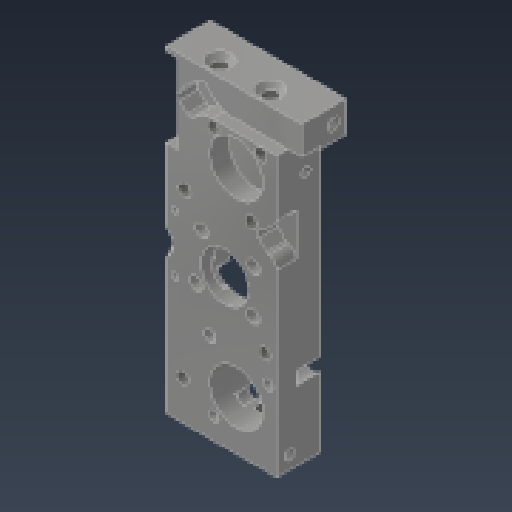
# Autodesk Inventor part: LeftGearbox
Saved by Autodesk Inventor 2027.1 (Build 311270010, 270A)
## iProperties
Created: 2026-04-13
Part Number: LeftGearbox
Material: Steel
Document SubType Name: Modeling
Designer: szymo
Density: 7.85 g/cm^3
Appearance: Nylon 6(1)
Mass: 68.9127 g
Surface Area: 68.8445 cm^2
Volume: 8.77869 cm^3
Author: szymo
Autodesk Inventor part; units mm, degrees
(part 1 of 2)
sketch "Sketch1" plane through (0, 0, 0) normal (0, 0, 1) x (1, 0, 0)
  circle A0 centre (14.75, -56.1789) radius 14.75 construction
  circle A1 centre (14.75, -56.1789) radius 14 construction
  circle A2 centre (14.75, -56.1789) radius 5.5
  circle A3 centre (14.7, -14.7) radius 5.5707
  circle A4 centre (14.7, -14.7) radius 14.7 construction
  circle A5 centre (12.35, -35.5681) radius 5
  circle A6 centre (9.3012, -47.7937) radius 8 construction
  circle A7 centre (9.3012, -47.7937) radius 4.2 construction
  circle A8 centre (12.35, -35.2722) radius 9.5572 construction
  line L0 (23.2, -66.4289) -> (0, -66.4289)
  line L1 (0, -66.4289) -> (0, 0)
  line L2 (0, 0) -> (23.2, 0)
  line L3 (23.2, 0) -> (23.2, -66.4289)
  circle A9 centre (12.35, -35.2722) radius 9.9572
  circle A10 centre (9.3012, -47.7937) radius 8.4
  line L4 (29.5, -56.1789) -> (23.2, -56.1789)
  line L5 (14.75, -56.1789) -> (23.2, -56.1789) construction
  line L6 (2.5, -8.5619) -> (2.3628, -10.4638) construction
  arc A11 (21.5927, -27.2496) -> (27.2496, -21.5927) centre (14.7, -14.7) ccw
  line L7 (27.2496, -21.5927) -> (24.0092, -18.3523)
  arc A12 (18.3523, -24.0092) -> (24.0092, -18.3523) centre (14.7, -14.7) ccw construction
  line L8 (18.3523, -24.0092) -> (21.5927, -27.2496)
  line L9 (18.3523, -24.0092) -> (24.0092, -18.3523)
  line L10 (23.2, -6.5) -> (28.4, -6.5)
  line L11 (28.4, -6.5) -> (28.4, 0)
  line L12 (28.4, 0) -> (23.2, 0)
  circle A13 centre (9.3012, -47.7937) radius 4.6
  circle A14 centre (14.75, -56.1789) radius 14.75 projected
  circle A15 centre (14.75, -56.1789) radius 14.25 projected
  circle A16 centre (9.0931, -61.8357) radius 1.0564 projected
  circle A17 centre (20.4069, -50.522) radius 1.0564 projected
  circle A18 centre (14.75, -56.1789) radius 5.5 projected
  circle A19 centre (14.75, -56.1789) radius 14.25 projected
  circle A20 centre (14.75, -14.75) radius 14.75 projected
  circle A21 centre (14.75, -14.75) radius 14.25 projected
  circle A22 centre (14.75, -14.75) radius 5.5 projected
  arc A23 (9.8338, -26.3037) -> (9.7739, -27.7306) centre (15.759, -27.2671) ccw projected
  arc A24 (10.3221, -26.1847) -> (9.8338, -26.3037) centre (12.35, -35.5681) ccw projected
  arc A25 (11.0317, -27.4241) -> (10.3221, -26.1847) centre (5.5043, -29.766) ccw projected
  arc A26 (11.4597, -27.3663) -> (11.0317, -27.4241) centre (12.35, -35.5681) ccw projected
  arc A27 (11.815, -25.983) -> (11.4597, -27.3663) centre (17.4104, -28.1572) ccw projected
  arc A28 (12.3173, -25.9682) -> (11.815, -25.983) centre (12.35, -35.5681) ccw projected
  arc A29 (12.7537, -27.328) -> (12.3173, -25.9682) centre (6.8602, -28.4694) ccw projected
  arc A30 (13.1844, -27.3604) -> (12.7537, -27.328) centre (12.35, -35.5681) ccw projected
  arc A31 (13.8195, -26.0813) -> (13.1844, -27.3604) centre (18.8407, -29.3713) ccw projected
  arc A32 (14.314, -26.1712) -> (13.8195, -26.0813) centre (12.35, -35.5681) ccw projected
  arc A33 (14.4581, -27.592) -> (14.314, -26.1712) centre (8.4561, -27.4832) ccw projected
  arc A34 (14.8727, -27.7133) -> (14.4581, -27.592) centre (12.35, -35.5681) ccw projected
  arc A35 (15.7598, -26.5941) -> (14.8727, -27.7133) centre (19.9872, -30.8562) ccw projected
  arc A36 (16.2248, -26.7848) -> (15.7598, -26.5941) centre (12.35, -35.5681) ccw projected
  arc A37 (16.0704, -28.2046) -> (16.2248, -26.7848) centre (10.2221, -26.8502) ccw projected
  arc A38 (16.4507, -28.4094) -> (16.0704, -28.2046) centre (12.35, -35.5681) ccw projected
  arc A39 (17.5511, -27.4991) -> (16.4507, -28.4094) centre (20.8, -32.547) ccw projected
  arc A40 (17.9663, -27.7824) -> (17.5511, -27.4991) centre (12.35, -35.5681) ccw projected
  arc A41 (17.52, -29.139) -> (17.9663, -27.7824) centre (12.0812, -26.5983) ccw projected
  arc A42 (17.8494, -29.4184) -> (17.52, -29.139) centre (12.35, -35.5681) ccw projected
  arc A43 (19.1151, -28.7568) -> (17.8494, -29.4184) centre (21.2434, -34.3699) ccw projected
  arc A44 (19.4623, -29.1202) -> (19.1151, -28.7568) centre (12.35, -35.5681) ccw projected
  arc A45 (18.7437, -30.3544) -> (19.4623, -29.1202) centre (13.952, -26.7385) ccw projected
  arc A46 (19.0078, -30.6962) -> (18.7437, -30.3544) centre (12.35, -35.5681) ccw projected
  arc A47 (20.3834, -30.3122) -> (19.0078, -30.6962) centre (21.2982, -36.2451) ccw projected
  arc A48 (20.6475, -30.7399) -> (20.3834, -30.3122) centre (12.35, -35.5681) ccw projected
  arc A49 (19.688, -31.7977) -> (20.6475, -30.7399) centre (15.7527, -27.2645) ccw projected
  arc A50 (19.8753, -32.1869) -> (19.688, -31.7977) centre (12.35, -35.5681) ccw projected
  arc A51 (21.3006, -32.0973) -> (19.8753, -32.1869) centre (20.9619, -38.0908) ccw projected
  arc A52 (21.47, -32.5705) -> (21.3006, -32.0973) centre (12.35, -35.5681) ccw projected
  arc A53 (20.3116, -33.4058) -> (21.47, -32.5705) centre (17.4048, -28.1534) ccw projected
  arc A54 (20.4138, -33.8254) -> (20.3116, -33.4058) centre (12.35, -35.5681) ccw projected
  arc A55 (21.8266, -34.0341) -> (20.4138, -33.8254) centre (20.2492, -39.8262) ccw projected
  arc A56 (21.8939, -34.5322) -> (21.8266, -34.0341) centre (12.35, -35.5681) ccw projected
  arc A57 (20.5872, -35.1083) -> (21.8939, -34.5322) centre (18.836, -29.3664) ccw projected
  arc A58 (20.6, -35.54) -> (20.5872, -35.1083) centre (12.35, -35.5681) ccw projected
  arc A59 (21.9385, -36.0379) -> (20.6, -35.54) centre (19.1913, -41.3755) ccw projected
  arc A60 (21.9008, -36.5391) -> (21.9385, -36.0379) centre (12.35, -35.5681) ccw projected
  arc A61 (20.5028, -36.831) -> (21.9008, -36.5391) centre (19.9836, -30.8504) ccw projected
  arc A62 (20.4255, -37.2559) -> (20.5028, -36.831) centre (12.35, -35.5681) ccw projected
  arc A63 (21.6313, -38.0212) -> (20.4255, -37.2559) centre (17.8344, -42.671) ccw projected
  arc A64 (21.4902, -38.5036) -> (21.6313, -38.0212) centre (12.35, -35.5681) ccw projected
  arc A65 (20.0621, -38.4984) -> (21.4902, -38.5036) centre (20.7977, -32.5406) ccw projected
  arc A66 (19.8981, -38.898) -> (20.0621, -38.4984) centre (12.35, -35.5681) ccw projected
  arc A67 (20.9184, -39.8973) -> (19.8981, -38.898) centre (16.2378, -43.656) ccw projected
  arc A68 (20.6801, -40.3398) -> (20.9184, -39.8973) centre (12.35, -35.5681) ccw projected
  arc A69 (19.2843, -40.0378) -> (20.6801, -40.3398) centre (21.2425, -34.3632) ccw projected
  arc A70 (19.0409, -40.3946) -> (19.2843, -40.0378) centre (12.35, -35.5681) ccw projected
  arc A71 (19.8311, -41.5842) -> (19.0409, -40.3946) centre (14.4713, -44.2876) ccw projected
  arc A72 (19.506, -41.9675) -> (19.8311, -41.5842) centre (12.35, -35.5681) ccw projected
  arc A73 (18.2034, -41.3819) -> (19.506, -41.9675) centre (21.2987, -36.2383) ccw projected
  arc A74 (17.8912, -41.6802) -> (18.2034, -41.3819) centre (12.35, -35.5681) ccw projected
  arc A75 (18.4168, -43.0081) -> (17.8912, -41.6802) centre (12.612, -44.5381) ccw projected
  arc A76 (18.0191, -43.3154) -> (18.4168, -43.0081) centre (12.35, -35.5681) ccw projected
  arc A77 (16.8668, -42.4718) -> (18.0191, -43.3154) centre (20.9638, -38.0842) ccw projected
  arc A78 (16.4993, -42.6987) -> (16.8668, -42.4718) centre (12.35, -35.5681) ccw projected
  arc A79 (16.7374, -44.1069) -> (16.4993, -42.6987) centre (10.7413, -44.3966) ccw projected
  arc A80 (16.2845, -44.3248) -> (16.7374, -44.1069) centre (12.35, -35.5681) ccw projected
  arc A81 (15.3327, -43.26) -> (16.2845, -44.3248) centre (20.2525, -39.8202) ccw projected
  arc A82 (14.9261, -43.4056) -> (15.3327, -43.26) centre (12.35, -35.5681) ccw projected
  arc A83 (14.8662, -44.8325) -> (14.9261, -43.4056) centre (8.941, -43.8692) ccw projected
  arc A84 (14.3779, -44.9515) -> (14.8662, -44.8325) centre (12.35, -35.5681) ccw projected
  arc A85 (13.6683, -43.7121) -> (14.3779, -44.9515) centre (19.1957, -41.3703) ccw projected
  arc A86 (13.2403, -43.7699) -> (13.6683, -43.7121) centre (12.35, -35.5681) ccw projected
  arc A87 (12.885, -45.1532) -> (13.2403, -43.7699) centre (7.2896, -42.979) ccw projected
  arc A88 (12.3827, -45.1681) -> (12.885, -45.1532) centre (12.35, -35.5681) ccw projected
  arc A89 (11.9463, -43.8082) -> (12.3827, -45.1681) centre (17.8398, -42.6668) ccw projected
  arc A90 (11.5156, -43.7758) -> (11.9463, -43.8082) centre (12.35, -35.5681) ccw projected
  arc A91 (10.8805, -45.055) -> (11.5156, -43.7758) centre (5.8593, -41.7649) ccw projected
  arc A92 (10.386, -44.9651) -> (10.8805, -45.055) centre (12.35, -35.5681) ccw projected
  arc A93 (10.2419, -43.5442) -> (10.386, -44.9651) centre (16.2439, -43.6531) ccw projected
  arc A94 (9.8273, -43.423) -> (10.2419, -43.5442) centre (12.35, -35.5681) ccw projected
  arc A95 (8.9402, -44.5421) -> (9.8273, -43.423) centre (4.7128, -40.28) ccw projected
  arc A96 (8.4752, -44.3514) -> (8.9402, -44.5421) centre (12.35, -35.5681) ccw projected
  arc A97 (8.6296, -42.9316) -> (8.4752, -44.3514) centre (14.4779, -44.286) ccw projected
  arc A98 (8.2493, -42.7268) -> (8.6296, -42.9316) centre (12.35, -35.5681) ccw projected
  arc A99 (7.1489, -43.6371) -> (8.2493, -42.7268) centre (3.9, -38.5892) ccw projected
  arc A100 (6.7337, -43.3538) -> (7.1489, -43.6371) centre (12.35, -35.5681) ccw projected
  arc A101 (7.18, -41.9972) -> (6.7337, -43.3538) centre (12.6188, -44.5379) ccw projected
  arc A102 (6.8506, -41.7178) -> (7.18, -41.9972) centre (12.35, -35.5681) ccw projected
  arc A103 (5.5849, -42.3794) -> (6.8506, -41.7178) centre (3.4566, -36.7663) ccw projected
  arc A104 (5.2377, -42.016) -> (5.5849, -42.3794) centre (12.35, -35.5681) ccw projected
  arc A105 (5.9563, -40.7818) -> (5.2377, -42.016) centre (10.748, -44.3978) ccw projected
  arc A106 (5.6922, -40.44) -> (5.9563, -40.7818) centre (12.35, -35.5681) ccw projected
  arc A107 (4.3166, -40.824) -> (5.6922, -40.44) centre (3.4018, -34.8911) ccw projected
  arc A108 (4.0525, -40.3964) -> (4.3166, -40.824) centre (12.35, -35.5681) ccw projected
  arc A109 (5.012, -39.3385) -> (4.0525, -40.3964) centre (8.9473, -43.8718) ccw projected
  arc A110 (4.8247, -38.9493) -> (5.012, -39.3385) centre (12.35, -35.5681) ccw projected
  arc A111 (3.3994, -39.0389) -> (4.8247, -38.9493) centre (3.7381, -33.0454) ccw projected
  arc A112 (3.23, -38.5657) -> (3.3994, -39.0389) centre (12.35, -35.5681) ccw projected
  arc A113 (4.3884, -37.7305) -> (3.23, -38.5657) centre (7.2952, -42.9828) ccw projected
  arc A114 (4.2862, -37.3108) -> (4.3884, -37.7305) centre (12.35, -35.5681) ccw projected
  arc A115 (2.8734, -37.1021) -> (4.2862, -37.3108) centre (4.4508, -31.31) ccw projected
  arc A116 (2.8061, -36.6041) -> (2.8734, -37.1021) centre (12.35, -35.5681) ccw projected
  arc A117 (4.1128, -36.0279) -> (2.8061, -36.6041) centre (5.864, -41.7699) ccw projected
  arc A118 (4.1, -35.5962) -> (4.1128, -36.0279) centre (12.35, -35.5681) ccw projected
  arc A119 (2.7615, -35.0983) -> (4.1, -35.5962) centre (5.5087, -29.7608) ccw projected
  arc A120 (2.7992, -34.5971) -> (2.7615, -35.0983) centre (12.35, -35.5681) ccw projected
  arc A121 (4.1972, -34.3053) -> (2.7992, -34.5971) centre (4.7164, -40.2858) ccw projected
  arc A122 (4.2745, -33.8803) -> (4.1972, -34.3053) centre (12.35, -35.5681) ccw projected
  arc A123 (3.0687, -33.115) -> (4.2745, -33.8803) centre (6.8656, -28.4653) ccw projected
  arc A124 (3.2098, -32.6326) -> (3.0687, -33.115) centre (12.35, -35.5681) ccw projected
  arc A125 (4.6379, -32.6378) -> (3.2098, -32.6326) centre (3.9023, -38.5956) ccw projected
  arc A126 (4.8019, -32.2382) -> (4.6379, -32.6378) centre (12.35, -35.5681) ccw projected
  arc A127 (3.7816, -31.2389) -> (4.8019, -32.2382) centre (8.4622, -27.4802) ccw projected
  arc A128 (4.0199, -30.7964) -> (3.7816, -31.2389) centre (12.35, -35.5681) ccw projected
  arc A129 (5.4157, -31.0984) -> (4.0199, -30.7964) centre (3.4575, -36.7731) ccw projected
  arc A130 (5.6591, -30.7416) -> (5.4157, -31.0984) centre (12.35, -35.5681) ccw projected
  arc A131 (4.8689, -29.5521) -> (5.6591, -30.7416) centre (10.2287, -26.8486) ccw projected
  arc A132 (5.194, -29.1688) -> (4.8689, -29.5521) centre (12.35, -35.5681) ccw projected
  arc A133 (6.4966, -29.7544) -> (5.194, -29.1688) centre (3.4013, -34.8979) ccw projected
  arc A134 (6.8088, -29.456) -> (6.4966, -29.7544) centre (12.35, -35.5681) ccw projected
  arc A135 (6.2832, -28.1281) -> (6.8088, -29.456) centre (12.088, -26.5981) ccw projected
  arc A136 (6.6809, -27.8208) -> (6.2832, -28.1281) centre (12.35, -35.5681) ccw projected
  arc A137 (7.8332, -28.6644) -> (6.6809, -27.8208) centre (3.7362, -33.052) ccw projected
  arc A138 (8.2007, -28.4375) -> (7.8332, -28.6644) centre (12.35, -35.5681) ccw projected
  arc A139 (7.9626, -27.0293) -> (8.2007, -28.4375) centre (13.9587, -26.7397) ccw projected
  arc A140 (8.4155, -26.8114) -> (7.9626, -27.0293) centre (12.35, -35.5681) ccw projected
  arc A141 (9.3673, -27.8762) -> (8.4155, -26.8114) centre (4.4475, -31.316) ccw projected
  arc A142 (9.7739, -27.7306) -> (9.3673, -27.8762) centre (12.35, -35.5681) ccw projected
  circle A143 centre (9.3012, -47.7937) radius 1.25 projected
  arc A144 (9.6251, -54.6611) -> (10.0958, -55.7541) centre (14.4225, -53.2431) ccw projected
  arc A145 (9.2653, -54.6686) -> (9.6251, -54.6611) centre (9.3012, -47.7937) ccw projected
  arc A146 (8.8408, -55.7804) -> (9.2653, -54.6686) centre (4.4127, -53.4528) ccw projected
  arc A147 (8.4234, -55.7454) -> (8.8408, -55.7804) centre (9.3012, -47.7937) ccw projected
  arc A148 (8.1902, -54.5783) -> (8.4234, -55.7454) centre (13.1776, -54.1888) ccw projected
  arc A149 (7.8367, -54.5109) -> (8.1902, -54.5783) centre (9.3012, -47.7937) ccw projected
  arc A150 (7.1903, -55.5102) -> (7.8367, -54.5109) centre (3.3429, -52.3128) ccw projected
  arc A151 (6.7893, -55.3891) -> (7.1903, -55.5102) centre (9.3012, -47.7937) ccw projected
  arc A152 (6.8039, -54.1991) -> (6.7893, -55.3891) centre (11.7633, -54.855) ccw projected
  arc A153 (6.4721, -54.0596) -> (6.8039, -54.1991) centre (9.3012, -47.7937) ccw projected
  arc A154 (5.6321, -54.9027) -> (6.4721, -54.0596) centre (2.5336, -50.9752) ccw projected
  arc A155 (5.265, -54.7009) -> (5.6321, -54.9027) centre (9.3012, -47.7937) ccw projected
  arc A156 (5.5267, -53.5399) -> (5.265, -54.7009) centre (10.2414, -55.2125) ccw projected
  arc A157 (5.2312, -53.3345) -> (5.5267, -53.5399) centre (9.3012, -47.7937) ccw projected
  arc A158 (4.2342, -53.9845) -> (5.2312, -53.3345) centre (2.02, -49.4986) ccw projected
  arc A159 (3.9172, -53.7108) -> (4.2342, -53.9845) centre (9.3012, -47.7937) ccw projected
  arc A160 (4.4145, -52.6296) -> (3.9172, -53.7108) centre (8.6783, -55.2459) ccw projected
  arc A161 (4.1681, -52.3672) -> (4.4145, -52.6296) centre (9.3012, -47.7937) ccw projected
  arc A162 (3.0578, -52.7957) -> (4.1681, -52.3672) centre (1.8246, -47.9475) ccw projected
  arc A163 (2.8046, -52.4621) -> (3.0578, -52.7957) centre (9.3012, -47.7937) ccw projected
  arc A164 (3.5159, -51.5079) -> (2.8046, -52.4621) centre (7.1426, -54.9535) ccw projected
  arc A165 (3.3294, -51.2) -> (3.5159, -51.5079) centre (9.3012, -47.7937) ccw projected
  arc A166 (2.1543, -51.3883) -> (3.3294, -51.2) centre (1.956, -46.3897) ccw projected
  arc A167 (1.9759, -51.0093) -> (2.1543, -51.3883) centre (9.3012, -47.7937) ccw projected
  arc A168 (2.8701, -50.2239) -> (1.9759, -51.0093) centre (5.7011, -54.3483) ccw projected
  arc A169 (2.7517, -49.884) -> (2.8701, -50.2239) centre (9.3012, -47.7937) ccw projected
  arc A170 (1.5631, -49.8238) -> (2.7517, -49.884) centre (2.4085, -44.8932) ccw projected
  arc A171 (1.4674, -49.4161) -> (1.5631, -49.8238) centre (9.3012, -47.7937) ccw projected
  arc A172 (2.5053, -48.8337) -> (1.4674, -49.4161) centre (4.417, -53.4565) ccw projected
  arc A173 (2.4602, -48.4766) -> (2.5053, -48.8337) centre (9.3012, -47.7937) ccw projected
  arc A174 (1.3101, -48.1706) -> (2.4602, -48.4766) centre (3.1621, -43.5235) ccw projected
  arc A175 (1.3013, -47.7519) -> (1.3101, -48.1706) centre (9.3012, -47.7937) ccw projected
  arc A176 (2.4376, -47.398) -> (1.3013, -47.7519) centre (3.3464, -52.3173) ccw projected
  arc A177 (2.4677, -47.0393) -> (2.4376, -47.398) centre (9.3012, -47.7937) ccw projected
  arc A178 (1.4064, -46.5009) -> (2.4677, -47.0393) centre (4.1841, -42.3404) ccw projected
  arc A179 (1.4848, -46.0895) -> (1.4064, -46.5009) centre (9.3012, -47.7937) ccw projected
  arc A180 (2.6699, -45.9796) -> (1.4848, -46.0895) centre (2.536, -50.9804) ccw projected
  arc A181 (2.7739, -45.635) -> (2.6699, -45.9796) centre (9.3012, -47.7937) ccw projected
  arc A182 (1.8477, -44.8877) -> (2.7739, -45.635) centre (5.4297, -41.3957) ccw projected
  arc A183 (2.01, -44.5016) -> (1.8477, -44.8877) centre (9.3012, -47.7937) ccw projected
  arc A184 (3.192, -44.6405) -> (2.01, -44.5016) centre (2.0213, -49.5042) ccw projected
  arc A185 (3.3653, -44.3251) -> (3.192, -44.6405) centre (9.3012, -47.7937) ccw projected
  arc A186 (2.6147, -43.4016) -> (3.3653, -44.3251) centre (6.8445, -40.7306) ccw projected
  arc A187 (2.8538, -43.0576) -> (2.6147, -43.4016) centre (9.3012, -47.7937) ccw projected
  arc A188 (3.981, -43.4392) -> (2.8538, -43.0576) centre (1.8248, -47.9532) ccw projected
  arc A189 (4.2162, -43.1668) -> (3.981, -43.4392) centre (9.3012, -47.7937) ccw projected
  arc A190 (3.674, -42.1073) -> (4.2162, -43.1668) centre (8.3667, -40.3741) ccw projected
  arc A191 (3.9793, -41.8206) -> (3.674, -42.1073) centre (9.3012, -47.7937) ccw projected
  arc A192 (5.0026, -42.4283) -> (3.9793, -41.8206) centre (1.955, -46.3953) ccw projected
  arc A193 (5.2893, -42.2107) -> (5.0026, -42.4283) centre (9.3012, -47.7937) ccw projected
  arc A194 (4.9792, -41.0616) -> (5.2893, -42.2107) centre (9.9298, -40.342) ccw projected
  arc A195 (5.3375, -40.8447) -> (4.9792, -41.0616) centre (9.3012, -47.7937) ccw projected
  arc A196 (6.2121, -41.6518) -> (5.3375, -40.8447) centre (2.4062, -44.8985) ccw projected
  arc A197 (6.5378, -41.4985) -> (6.2121, -41.6518) centre (9.3012, -47.7937) ccw projected
  arc A198 (6.4734, -40.3102) -> (6.5378, -41.4985) centre (11.4653, -40.6355) ccw projected
  arc A199 (6.8689, -40.1724) -> (6.4734, -40.3102) centre (9.3012, -47.7937) ccw projected
  arc A200 (7.5566, -41.1437) -> (6.8689, -40.1724) centre (3.1589, -43.5282) ccw projected
  arc A201 (7.907, -41.0616) -> (7.5566, -41.1437) centre (9.3012, -47.7937) ccw projected
  arc A202 (8.0911, -39.8858) -> (7.907, -41.0616) centre (12.9063, -41.2419) ccw projected
  arc A203 (8.5066, -39.8333) -> (8.0911, -39.8858) centre (9.3012, -47.7937) ccw projected
  arc A204 (8.9773, -40.9263) -> (8.5066, -39.8333) centre (4.18, -42.3443) ccw projected
  arc A205 (9.3372, -40.9188) -> (8.9773, -40.9263) centre (9.3012, -47.7937) ccw projected
  arc A206 (9.7617, -39.807) -> (9.3372, -40.9188) centre (14.1897, -42.1346) ccw projected
  arc A207 (10.179, -39.842) -> (9.7617, -39.807) centre (9.3012, -47.7937) ccw projected
  arc A208 (10.4122, -41.0091) -> (10.179, -39.842) centre (5.4249, -41.3986) ccw projected
  arc A209 (10.7658, -41.0765) -> (10.4122, -41.0091) centre (9.3012, -47.7937) ccw projected
  arc A210 (11.4121, -40.0772) -> (10.7658, -41.0765) centre (15.2595, -43.2746) ccw projected
  arc A211 (11.8131, -40.1983) -> (11.4121, -40.0772) centre (9.3012, -47.7937) ccw projected
  arc A212 (11.7985, -41.3883) -> (11.8131, -40.1983) centre (6.8392, -40.7324) ccw projected
  arc A213 (12.1303, -41.5278) -> (11.7985, -41.3883) centre (9.3012, -47.7937) ccw projected
  arc A214 (12.9704, -40.6847) -> (12.1303, -41.5278) centre (16.0689, -44.6122) ccw projected
  arc A215 (13.3374, -40.8865) -> (12.9704, -40.6847) centre (9.3012, -47.7937) ccw projected
  arc A216 (13.0757, -42.0475) -> (13.3374, -40.8865) centre (8.3611, -40.3749) ccw projected
  arc A217 (13.3713, -42.2529) -> (13.0757, -42.0475) centre (9.3012, -47.7937) ccw projected
  arc A218 (14.3682, -41.6029) -> (13.3713, -42.2529) centre (16.5824, -46.0888) ccw projected
  arc A219 (14.6853, -41.8766) -> (14.3682, -41.6029) centre (9.3012, -47.7937) ccw projected
  arc A220 (14.1879, -42.9578) -> (14.6853, -41.8766) centre (9.9241, -40.3415) ccw projected
  arc A221 (14.4343, -43.2202) -> (14.1879, -42.9578) centre (9.3012, -47.7937) ccw projected
  arc A222 (15.5446, -42.7917) -> (14.4343, -43.2202) centre (16.7778, -47.6399) ccw projected
  arc A223 (15.7979, -43.1253) -> (15.5446, -42.7917) centre (9.3012, -47.7937) ccw projected
  arc A224 (15.0866, -44.0795) -> (15.7979, -43.1253) centre (11.4599, -40.6339) ccw projected
  arc A225 (15.273, -44.3874) -> (15.0866, -44.0795) centre (9.3012, -47.7937) ccw projected
  arc A226 (16.4482, -44.1991) -> (15.273, -44.3874) centre (16.6464, -49.1977) ccw projected
  arc A227 (16.6265, -44.5781) -> (16.4482, -44.1991) centre (9.3012, -47.7937) ccw projected
  arc A228 (15.7324, -45.3635) -> (16.6265, -44.5781) centre (12.9013, -41.2391) ccw projected
  arc A229 (15.8508, -45.7034) -> (15.7324, -45.3635) centre (9.3012, -47.7937) ccw projected
  arc A230 (17.0393, -45.7636) -> (15.8508, -45.7034) centre (16.194, -50.6942) ccw projected
  arc A231 (17.135, -46.1713) -> (17.0393, -45.7636) centre (9.3012, -47.7937) ccw projected
  arc A232 (16.0971, -46.7537) -> (17.135, -46.1713) centre (14.1854, -42.1309) ccw projected
  arc A233 (16.1422, -47.1108) -> (16.0971, -46.7537) centre (9.3012, -47.7937) ccw projected
  arc A234 (17.2923, -47.4168) -> (16.1422, -47.1108) centre (15.4403, -52.0639) ccw projected
  arc A235 (17.3011, -47.8355) -> (17.2923, -47.4168) centre (9.3012, -47.7937) ccw projected
  arc A236 (16.1648, -48.1894) -> (17.3011, -47.8355) centre (15.2561, -43.2701) ccw projected
  arc A237 (16.1347, -48.5481) -> (16.1648, -48.1894) centre (9.3012, -47.7937) ccw projected
  arc A238 (17.1961, -49.0865) -> (16.1347, -48.5481) centre (14.4183, -53.247) ccw projected
  arc A239 (17.1176, -49.4979) -> (17.1961, -49.0865) centre (9.3012, -47.7937) ccw projected
  arc A240 (15.9326, -49.6078) -> (17.1176, -49.4979) centre (16.0664, -44.607) ccw projected
  arc A241 (15.8285, -49.9524) -> (15.9326, -49.6078) centre (9.3012, -47.7937) ccw projected
  arc A242 (16.7548, -50.6997) -> (15.8285, -49.9524) centre (13.1727, -54.1917) ccw projected
  arc A243 (16.5925, -51.0858) -> (16.7548, -50.6997) centre (9.3012, -47.7937) ccw projected
  arc A244 (15.4105, -50.9469) -> (16.5925, -51.0858) centre (16.5811, -46.0832) ccw projected
  arc A245 (15.2371, -51.2623) -> (15.4105, -50.9469) centre (9.3012, -47.7937) ccw projected
  arc A246 (15.9877, -52.1858) -> (15.2371, -51.2623) centre (11.7579, -54.8568) ccw projected
  arc A247 (15.7487, -52.5298) -> (15.9877, -52.1858) centre (9.3012, -47.7937) ccw projected
  arc A248 (14.6214, -52.1482) -> (15.7487, -52.5298) centre (16.7777, -47.6342) ccw projected
  arc A249 (14.3862, -52.4206) -> (14.6214, -52.1482) centre (9.3012, -47.7937) ccw projected
  arc A250 (14.9284, -53.4801) -> (14.3862, -52.4206) centre (10.2357, -55.2133) ccw projected
  arc A251 (14.6231, -53.7668) -> (14.9284, -53.4801) centre (9.3012, -47.7937) ccw projected
  arc A252 (13.5998, -53.1591) -> (14.6231, -53.7668) centre (16.6475, -49.1921) ccw projected
  arc A253 (13.3131, -53.3767) -> (13.5998, -53.1591) centre (9.3012, -47.7937) ccw projected
  arc A254 (13.6232, -54.5258) -> (13.3131, -53.3767) centre (8.6727, -55.2454) ccw projected
  arc A255 (13.2649, -54.7427) -> (13.6232, -54.5258) centre (9.3012, -47.7937) ccw projected
  arc A256 (12.3903, -53.9356) -> (13.2649, -54.7427) centre (16.1962, -50.6889) ccw projected
  arc A257 (12.0647, -54.0889) -> (12.3903, -53.9356) centre (9.3012, -47.7937) ccw projected
  arc A258 (12.1291, -55.2772) -> (12.0647, -54.0889) centre (7.1371, -54.9519) ccw projected
  arc A259 (11.7335, -55.415) -> (12.1291, -55.2772) centre (9.3012, -47.7937) ccw projected
  arc A260 (11.0459, -54.4437) -> (11.7335, -55.415) centre (15.4436, -52.0592) ccw projected
  arc A261 (10.6954, -54.5258) -> (11.0459, -54.4437) centre (9.3012, -47.7937) ccw projected
  arc A262 (10.5114, -55.7016) -> (10.6954, -54.5258) centre (5.6961, -54.3455) ccw projected
  arc A263 (10.0958, -55.7541) -> (10.5114, -55.7016) centre (9.3012, -47.7937) ccw projected
  circle A264 centre (9.3012, -47.7937) radius 1.25 projected
  arc A265 (10.3711, -45.1522) -> (10.3563, -43.7284) centre (6.7284, -44.4781) ccw projected
  arc A266 (10.7068, -45.3144) -> (10.3711, -45.1522) centre (9.3012, -47.7937) ccw projected
  arc A267 (11.8317, -44.4416) -> (10.7068, -45.3144) centre (13.4977, -47.7504) ccw projected
  arc A268 (12.2476, -44.8006) -> (11.8317, -44.4416) centre (9.3012, -47.7937) ccw projected
  arc A269 (11.5486, -46.041) -> (12.2476, -44.8006) centre (8.7309, -43.6359) ccw projected
  arc A270 (11.7581, -46.3493) -> (11.5486, -46.041) centre (9.3012, -47.7937) ccw projected
  arc A271 (13.1688, -46.156) -> (11.7581, -46.3493) centre (12.9572, -49.8545) ccw projected
  arc A272 (13.3494, -46.6748) -> (13.1688, -46.156) centre (9.3012, -47.7937) ccw projected
  arc A273 (12.1238, -47.3995) -> (13.3494, -46.6748) centre (10.8863, -43.9078) ccw projected
  arc A274 (12.1511, -47.7713) -> (12.1238, -47.3995) centre (9.3012, -47.7937) ccw projected
  arc A275 (13.4695, -48.3092) -> (12.1511, -47.7713) centre (11.437, -51.4064) ccw projected
  arc A276 (13.3665, -48.8488) -> (13.4695, -48.3092) centre (9.3012, -47.7937) ccw projected
  arc A277 (11.9428, -48.8636) -> (13.3665, -48.8488) centre (12.6169, -45.2209) ccw projected
  arc A278 (11.7805, -49.1993) -> (11.9428, -48.8636) centre (9.3012, -47.7937) ccw projected
  arc A279 (12.6533, -50.3242) -> (11.7805, -49.1993) centre (9.3445, -51.9902) ccw projected
  arc A280 (12.2943, -50.7401) -> (12.6533, -50.3242) centre (9.3012, -47.7937) ccw projected
  arc A281 (11.0539, -50.041) -> (12.2943, -50.7401) centre (13.459, -47.2234) ccw projected
  arc A282 (10.7456, -50.2506) -> (11.0539, -50.041) centre (9.3012, -47.7937) ccw projected
  arc A283 (10.9389, -51.6612) -> (10.7456, -50.2506) centre (7.2404, -51.4496) ccw projected
  arc A284 (10.4201, -51.8419) -> (10.9389, -51.6612) centre (9.3012, -47.7937) ccw projected
  arc A285 (9.6954, -50.6163) -> (10.4201, -51.8419) centre (13.1871, -49.3787) ccw projected
  arc A286 (9.3236, -50.6436) -> (9.6954, -50.6163) centre (9.3012, -47.7937) ccw projected
  arc A287 (8.7858, -51.9619) -> (9.3236, -50.6436) centre (5.6886, -49.9294) ccw projected
  arc A288 (8.2461, -51.859) -> (8.7858, -51.9619) centre (9.3012, -47.7937) ccw projected
  arc A289 (8.2313, -50.4352) -> (8.2461, -51.859) centre (11.874, -51.1093) ccw projected
  arc A290 (7.8957, -50.273) -> (8.2313, -50.4352) centre (9.3012, -47.7937) ccw projected
  arc A291 (6.7707, -51.1458) -> (7.8957, -50.273) centre (5.1047, -47.837) ccw projected
  arc A292 (6.3548, -50.7868) -> (6.7707, -51.1458) centre (9.3012, -47.7937) ccw projected
  arc A293 (7.0539, -49.5464) -> (6.3548, -50.7868) centre (9.8715, -51.9515) ccw projected
  arc A294 (6.8443, -49.2381) -> (7.0539, -49.5464) centre (9.3012, -47.7937) ccw projected
  arc A295 (5.4337, -49.4314) -> (6.8443, -49.2381) centre (5.6453, -45.7329) ccw projected
  arc A296 (5.253, -48.9126) -> (5.4337, -49.4314) centre (9.3012, -47.7937) ccw projected
  arc A297 (6.4786, -48.1879) -> (5.253, -48.9126) centre (7.7162, -51.6796) ccw projected
  arc A298 (6.4513, -47.8161) -> (6.4786, -48.1879) centre (9.3012, -47.7937) ccw projected
  arc A299 (5.133, -47.2782) -> (6.4513, -47.8161) centre (7.1655, -44.181) ccw projected
  arc A300 (5.2359, -46.7386) -> (5.133, -47.2782) centre (9.3012, -47.7937) ccw projected
  arc A301 (6.6597, -46.7238) -> (5.2359, -46.7386) centre (5.9856, -50.3665) ccw projected
  arc A302 (6.8219, -46.3881) -> (6.6597, -46.7238) centre (9.3012, -47.7937) ccw projected
  arc A303 (5.9491, -45.2632) -> (6.8219, -46.3881) centre (9.2579, -43.5972) ccw projected
  arc A304 (6.3081, -44.8473) -> (5.9491, -45.2632) centre (9.3012, -47.7937) ccw projected
  arc A305 (7.5485, -45.5464) -> (6.3081, -44.8473) centre (5.1434, -48.364) ccw projected
  arc A306 (7.8569, -45.3368) -> (7.5485, -45.5464) centre (9.3012, -47.7937) ccw projected
  arc A307 (7.6635, -43.9262) -> (7.8569, -45.3368) centre (11.362, -44.1378) ccw projected
  arc A308 (8.1823, -43.7455) -> (7.6635, -43.9262) centre (9.3012, -47.7937) ccw projected
  arc A309 (8.907, -44.9711) -> (8.1823, -43.7455) centre (5.4153, -46.2087) ccw projected
  arc A310 (9.2788, -44.9438) -> (8.907, -44.9711) centre (9.3012, -47.7937) ccw projected
  arc A311 (9.8167, -43.6255) -> (9.2788, -44.9438) centre (12.9139, -45.658) ccw projected
  arc A312 (10.3563, -43.7284) -> (9.8167, -43.6255) centre (9.3012, -47.7937) ccw projected
  circle A313 centre (12.35, -35.2722) radius 4.8 construction
  line L13 (2.5, -1) -> (1, -1)
  line L14 (1, -1) -> (1, -17.5)
  line L15 (1, -17.5) -> (2.5, -17.5)
  line L16 (2.5, -17.5) -> (2.5, -1)
  line L17 (1.5, -1) -> (1.5, -17) projected
  line L18 (2.5, -1) -> (1.5, -1) projected
  line L19 (2.5, -17) -> (2.5, -1) projected
  line L20 (2.5, -17) -> (1.5, -17) projected
  line L21 (1, -17.5) -> (0, -17.5)
  line L22 (1, -1) -> (0, -1)
  line L23 (26.7043, -21.0474) -> (25.0617, -19.4049) projected
  arc A314 (25.0617, -19.4049) -> (23.4815, -19.6245) centre (24.3546, -20.112) ccw projected
  arc A315 (19.6245, -23.4815) -> (23.4815, -19.6245) centre (14.75, -14.75) ccw projected
  arc A316 (19.6245, -23.4815) -> (19.4049, -25.0617) centre (20.112, -24.3546) ccw projected
  line L24 (19.4049, -25.0617) -> (21.0474, -26.7043) projected
  arc A317 (21.0474, -26.7043) -> (22.2832, -26.846) centre (21.7545, -25.9972) ccw projected
  arc A318 (2.654, -7.2168) -> (22.2832, -26.846) centre (14.75, -14.75) ccw projected
  arc A319 (2.654, -7.2168) -> (2.7957, -8.4526) centre (3.5028, -7.7455) ccw projected
  line L25 (2.7957, -8.4526) -> (4.4383, -10.0951) projected
  arc A320 (4.4383, -10.0951) -> (6.0185, -9.8755) centre (5.1454, -9.388) ccw projected
  arc A321 (9.8755, -6.0185) -> (6.0185, -9.8755) centre (14.75, -14.75) ccw projected
  arc A322 (9.8755, -6.0185) -> (10.0951, -4.4383) centre (9.388, -5.1454) ccw projected
  line L26 (10.0951, -4.4383) -> (8.4526, -2.7957) projected
  arc A323 (8.4526, -2.7957) -> (7.2168, -2.654) centre (7.7455, -3.5028) ccw projected
  arc A324 (26.846, -22.2832) -> (7.2168, -2.654) centre (14.75, -14.75) ccw projected
  arc A325 (26.846, -22.2832) -> (26.7043, -21.0474) centre (25.9972, -21.7545) ccw projected
  line L27 (7.2556, -8.1293) -> (23.2, -8.1293)
  line L28 (9.7861, -4.1293) -> (23.2, -4.1293)
  point P0 (0, 0)
  point P1 (23.2, -9.2314)
  point P2 (4.2588, -41.0755)
  point P3 (16.8677, -44.1456)
  point P4 (13.3936, -40.458)
  point P5 (9.1326, -39.3954)
  point P6 (13.101, -45.201)
  point P7 (7.1187, -43.7444)
  point P8 (16.9976, -51.1591)
  point P9 (9.25, -56.1935)
  point P10 (6.8877, -8.4575)
  point P11 (5.3877, -11.0556)
  point P12 (24.0123, -18.3444)
  point P13 (22.5123, -20.9425)
  point P14 (0.2586, -17.5)
  point P15 (0, -14.75)
  point P16 (1, -1)
  point P17 (9.9295, -39.4172)
  point P18 (12.594, -40.066)
  dimension "d0" = 4.5
  dimension "d2" = 0.4
  dimension "d3" = 0.4
  dimension "d5" = 6.3
  dimension "d8" = 1
  dimension "d10" = 0.4
  dimension "d19" = 10
  dimension "d56" = 0.5
  dimension "d57" = 0.5
  dimension "d77" = 0
  dimension "d78" = 0
  dimension "d156" = 6.5
  dimension "d253" = 1
  dimension "d254" = 4
  constraints: 42 end point, 13 point on line, 10 centre point, 9 coincident, 9 perpendicular, 5 point on circle, 5 tangent, 4 collinear, 4 parallel, 2 horizontal, 2 horizontal alignment, 19 other
  measures "d5" distance of L4.start L4.end
  measures "d8" distance edge to line of A4 L11
  measures "d19" diameter of A5
  measures "d56" distance between parallel lines of L14 L17
  measures "d57" distance between parallel lines of L15 L20
  measures "d77" distance between parallel lines of L18 L22
  measures "d78" distance between parallel lines of L15 L21
  measures "d156" distance between parallel lines of L10 L12
  measures "d253" distance edge to line of A3 L27
  measures "d254" distance between parallel lines of L27 L28
extrude "Extrusion1" add sketch "Sketch1" against normal blind 1.6 contours A2 A10 A9 A15 L3 L0 | A2 A243 A242 A241 A240 A239 A238 A237 A236 A235 A234 A233 A232 A231 A230 A229 A228 A227 A9 A10 | A10 A15 A170 A169 A168 A167 A166 A165 A164 A163 A162 A161 A160 A159 A158 A157 A156 A155 A154 A153 A152 A151 A150 A149 A148 A147 A146 A145 A2 | A2 A13 A9 A227 A228 A229 A230 A231 A232 A233 A234 A235 A236 A237 A238 A239 A240 A241 A242 A243 | A145 A146 A147 A148 A149 A150 A151 A152 A153 A154 A155 A156 A157 A158 A159 A160 A161 A162 A163 A164 A165 A166 A167 A168 A169 A170 A15 A13 A2 | A15 L0 A14 A10 | A10 A14 A171 A170 A15 | A2 A13 A15 A9 A307 A306 A305 A304 A303 A302 A301 A300 A299 A298 A297 A296 A295 A294 A293 A292 A291 A290 A289 A288 A287 A286 A285 A284 A283 A282 A281 A280 A279 A278 A277 A276 A275 A274 A273 A272 A271 A270 A269 | A10 A79 A78 A77 A76 A75 A15 A9 | A9 A227 A80 A79 A10 | A14 L1 L21 A20 A9 A10 | A10 A9 A193 A192 A191 A190 A189 A188 A187 A186 A185 A184 A183 A182 A181 A180 A179 A178 A177 A176 A175 A174 A14 A172 A171 | A170 A171 A14 A172 A173 A174 A9 A13 A15 | A9 A13 A87 A86 A85 A84 A83 A82 A81 A224 A225 A226 A80 A227 | A15 A75 A14 A9 | A9 A14 L3 A15 | A79 A80 A227 A226 A81 A224 A223 A222 A221 A220 A15 A10 | A10 A15 A75 A76 A77 A78 A79 | A13 A9 A15 | A10 A107 A106 A105 A196 A195 A194 A193 A9 | A9 A20 A139 A138 A137 A136 A135 A134 A133 A132 A131 A130 A129 A128 A127 A126 A125 A124 A123 A122 A121 A120 A119 A118 A117 A116 A115 A114 A113 A112 A111 A110 A109 A108 A107 A10 | A171 A172 A14 | A14 L0 L1 | A9 A269 A89 A88 A87 A13 | A80 A81 A226 A227 | A14 A75 A74 A73 A72 A71 A70 A69 A68 A67 A66 A65 A64 A63 A62 A61 A60 A59 A58 A57 A56 A55 A54 A53 A52 A51 A50 A49 A48 A47 A46 A45 A44 A20 A9 | A9 A20 L3 A14 | A15 A10 A14 A75 | A15 A220 A219 A218 A216 A14 A10 | A13 A97 A15 A9 | A9 A14 A100 A99 A98 A97 A13 | A15 A97 A309 A308 A307 A9 | A20 L21 A21 A9 | A9 A21 A139 A20 | A193 A194 A195 A196 A105 A104 A103 A102 A101 A100 A14 A9 | A9 A14 A174 A175 A176 A177 A178 A179 A180 A181 A182 A183 A184 A185 A186 A187 A188 A189 A190 A191 A192 A193 | A107 A108 A109 A110 A111 A112 A113 A114 A115 A116 A117 A118 A119 A120 A121 A122 A123 A124 A125 A126 A127 A128 A129 A130 A131 A132 A133 A134 A135 A136 A137 A138 A139 A20 A42 A43 A44 A45 A46 A47 A48 A49 A50 A51 A52 A53 A54 A55 A56 A57 A58 A59 A60 A61 A62 A63 A64 A65 A66 A67 A68 A69 A70 A71 A72 A73 A74 A75 A14 A10 A5 | A10 A5 A206 A205 A204 A203 A202 A201 A200 A199 A198 A197 A196 A105 A106 A107 | A14 A174 A173 A172 | A269 A270 A271 A272 A273 A274 A275 A276 A277 A278 A279 A280 A281 A282 A283 A284 A285 A286 A287 A288 A289 A290 A291 A292 A293 A294 A295 A296 A297 A298 A299 A300 A301 A302 A303 A304 A305 A306 A307 A9 A309 A310 A311 A265 A266 A267 | A9 A267 A268 A89 A269 | A87 A88 A89 A269 A268 A13 | A13 A89 A90 A15 A216 A217 A218 A220 A221 A222 A223 A224 A81 A82 A83 A84 A85 A86 A87 | A14 A216 A215 A214 A213 A212 A5 A10 | A15 A218 A219 A220 | A97 A98 A14 A216 A15 A13 | A13 A15 A97 | A307 A308 A309 A97 A96 A9 | A15 A13 A90 A91 A92 A265 A312 A93 A94 A95 A96 A309 A97 | A21 L21 L15 L16 A319 L25 A320 A321 L27 L3 L9 L8 A9 | A9 A21 A41 A40 A39 A38 A37 A36 A35 A34 A33 A32 A31 A30 A29 A28 A27 A26 A25 A24 A23 A142 A141 A140 A139 | A139 A21 A41 A42 A20 | A267 A266 A265 A9 | A9 A265 A92 A91 A90 A13 A89 A268 A267 | A89 A268 A269 | A13 A90 A89 | A226 A225 A224 A81 | A20 A44 A43 A42 A41 A21 A9 | A9 A21 A11 L3 A20 | A14 A98 A99 A100 A101 A102 A103 A104 A105 A196 A197 A198 A199 A200 A201 A202 A203 A204 A205 A206 A5 A208 A209 A210 A212 A213 A214 A215 A216 | A218 A217 A216 A15 | A14 A99 A100 | A309 A96 A95 A94 A93 A312 A311 A9 | A9 A311 A310 A309 | A309 A96 A97 | A139 A140 A141 A142 A23 A24 A25 A26 A27 A28 A29 A30 A31 A32 A33 A34 A35 A36 A37 A38 A39 A40 A41 A21 | A20 A43 A42 | L1 L2 A20 L16 L13 L22 | A9 A311 A312 A93 A92 A265 | A20 A43 A44 | A11 A317 L8 A316 A315 L3 | A14 A99 A98 | L8 A317 A11 | A5 A210 A209 A208 | A92 A93 A312 A265 | A315 A316 L8 L9 L3 | A20 L3 L12 L11 L10 | L10 A21 L3 A20 | L2 L3 A20 | A20 L3 A21 L16 | L10 L3 A21 | L27 A321 A322 L26 L28 L3 | L3 L28 L26 A323 A21 | A21 A323 L26 A322 A321 A320 L25 A319 | A22 | A3 | A16 | A17
extrude "Extrusion2" add sketch "Sketch1" against normal blind 3.1 contours A2 A10 A9 A15 L3 L0 | A2 A243 A242 A241 A240 A239 A238 A237 A236 A235 A234 A233 A232 A231 A230 A229 A228 A227 A9 A10 | A10 A15 A170 A169 A168 A167 A166 A165 A164 A163 A162 A161 A160 A159 A158 A157 A156 A155 A154 A153 A152 A151 A150 A149 A148 A147 A146 A145 A2 | A2 A13 A9 A227 A228 A229 A230 A231 A232 A233 A234 A235 A236 A237 A238 A239 A240 A241 A242 A243 | A145 A146 A147 A148 A149 A150 A151 A152 A153 A154 A155 A156 A157 A158 A159 A160 A161 A162 A163 A164 A165 A166 A167 A168 A169 A170 A15 A13 A2 | A15 L0 A14 A10 | A10 A14 A171 A170 A15 | A10 A79 A78 A77 A76 A75 A15 A9 | A9 A227 A80 A79 A10 | A14 L1 L21 A20 A9 A10 | A10 A9 A193 A192 A191 A190 A189 A188 A187 A186 A185 A184 A183 A182 A181 A180 A179 A178 A177 A176 A175 A174 A14 A172 A171 | A170 A171 A14 A172 A173 A174 A9 A13 A15 | A9 A13 A87 A86 A85 A84 A83 A82 A81 A224 A225 A226 A80 A227 | A15 A75 A14 A9 | A9 A14 L3 A15 | A79 A80 A227 A226 A81 A224 A223 A222 A221 A220 A15 A10 | A10 A15 A75 A76 A77 A78 A79 | A10 A107 A106 A105 A196 A195 A194 A193 A9 | A9 A20 A139 A138 A137 A136 A135 A134 A133 A132 A131 A130 A129 A128 A127 A126 A125 A124 A123 A122 A121 A120 A119 A118 A117 A116 A115 A114 A113 A112 A111 A110 A109 A108 A107 A10 | A171 A172 A14 | A14 L0 L1 | A80 A81 A226 A227 | A14 A75 A74 A73 A72 A71 A70 A69 A68 A67 A66 A65 A64 A63 A62 A61 A60 A59 A58 A57 A56 A55 A54 A53 A52 A51 A50 A49 A48 A47 A46 A45 A44 A20 A9 | A9 A20 L3 A14 | A15 A10 A14 A75 | A15 A220 A219 A218 A216 A14 A10 | A9 A14 A100 A99 A98 A97 A13 | A20 L21 A21 A9 | A9 A21 A139 A20 | A193 A194 A195 A196 A105 A104 A103 A102 A101 A100 A14 A9 | A9 A14 A174 A175 A176 A177 A178 A179 A180 A181 A182 A183 A184 A185 A186 A187 A188 A189 A190 A191 A192 A193 | A107 A108 A109 A110 A111 A112 A113 A114 A115 A116 A117 A118 A119 A120 A121 A122 A123 A124 A125 A126 A127 A128 A129 A130 A131 A132 A133 A134 A135 A136 A137 A138 A139 A20 A42 A43 A44 A45 A46 A47 A48 A49 A50 A51 A52 A53 A54 A55 A56 A57 A58 A59 A60 A61 A62 A63 A64 A65 A66 A67 A68 A69 A70 A71 A72 A73 A74 A75 A14 A10 A5 | A10 A5 A206 A205 A204 A203 A202 A201 A200 A199 A198 A197 A196 A105 A106 A107 | A14 A174 A173 A172 | A13 A89 A90 A15 A216 A217 A218 A220 A221 A222 A223 A224 A81 A82 A83 A84 A85 A86 A87 | A14 A216 A215 A214 A213 A212 A5 A10 | A15 A218 A219 A220 | A97 A98 A14 A216 A15 A13 | A21 L21 L15 L16 A319 L25 A320 A321 L27 L3 L9 L8 A9 | A9 A21 A41 A40 A39 A38 A37 A36 A35 A34 A33 A32 A31 A30 A29 A28 A27 A26 A25 A24 A23 A142 A141 A140 A139 | A139 A21 A41 A42 A20 | A13 A90 A89 | A226 A225 A224 A81 | A20 A44 A43 A42 A41 A21 A9 | A9 A21 A11 L3 A20 | A14 A98 A99 A100 A101 A102 A103 A104 A105 A196 A197 A198 A199 A200 A201 A202 A203 A204 A205 A206 A5 A208 A209 A210 A212 A213 A214 A215 A216 | A218 A217 A216 A15 | A14 A99 A100 | A139 A140 A141 A142 A23 A24 A25 A26 A27 A28 A29 A30 A31 A32 A33 A34 A35 A36 A37 A38 A39 A40 A41 A21 | A20 A43 A42 | L1 L2 A20 L16 L13 L22 | A20 A43 A44 | A11 A317 L8 A316 A315 L3 | A14 A99 A98 | L8 A317 A11 | A5 A210 A209 A208 | A315 A316 L8 L9 L3 | A20 L3 L12 L11 L10 | L10 A21 L3 A20 | L2 L3 A20 | A20 L3 A21 L16 | L10 L3 A21 | L27 A321 A322 L26 L28 L3 | L3 L28 L26 A323 A21 | A21 A323 L26 A322 A321 A320 L25 A319 | A22 | A3 | A16 | A17
extrude "Extrusion3" add sketch "Sketch1" against normal blind 6.2 contours A2 A10 A9 A15 L3 L0 | A2 A243 A242 A241 A240 A239 A238 A237 A236 A235 A234 A233 A232 A231 A230 A229 A228 A227 A9 A10 | A10 A15 A170 A169 A168 A167 A166 A165 A164 A163 A162 A161 A160 A159 A158 A157 A156 A155 A154 A153 A152 A151 A150 A149 A148 A147 A146 A145 A2 | A2 A13 A9 A227 A228 A229 A230 A231 A232 A233 A234 A235 A236 A237 A238 A239 A240 A241 A242 A243 | A145 A146 A147 A148 A149 A150 A151 A152 A153 A154 A155 A156 A157 A158 A159 A160 A161 A162 A163 A164 A165 A166 A167 A168 A169 A170 A15 A13 A2 | A15 L0 A14 A10 | A10 A14 A171 A170 A15 | A14 L1 L21 A20 A9 A10 | A10 A9 A193 A192 A191 A190 A189 A188 A187 A186 A185 A184 A183 A182 A181 A180 A179 A178 A177 A176 A175 A174 A14 A172 A171 | A170 A171 A14 A172 A173 A174 A9 A13 A15 | A9 A14 L3 A15 | A171 A172 A14 | A14 L0 L1 | A9 A20 L3 A14 | A20 L21 A21 A9 | A9 A14 A174 A175 A176 A177 A178 A179 A180 A181 A182 A183 A184 A185 A186 A187 A188 A189 A190 A191 A192 A193 | A14 A174 A173 A172 | A21 L21 L15 L16 A319 L25 A320 A321 L27 L3 L9 L8 A9 | A9 A21 A11 L3 A20 | L1 L2 A20 L16 L13 L22 | A11 A317 L8 A316 A315 L3 | L8 A317 A11 | A315 A316 L8 L9 L3 | A20 L3 L12 L11 L10 | L10 A21 L3 A20 | L2 L3 A20 | A20 L3 A21 L16 | L10 L3 A21 | L27 A321 A322 L26 L28 L3 | L3 L28 L26 A323 A21 | A21 A323 L26 A322 A321 A320 L25 A319 | A22 | A3 | A16 | A17
ref_plane "Work Plane1" through (6.5814, -41.0408, -9.3) normal (0, 0, -1) x (0.0707652, 0.997493, 0)
extrude "Extrusion4" add sketch "Sketch1" against normal up to surface (9.3 mm away) contours A2 A10 A9 A15 L3 L0 | A15 L0 A14 A10 | A14 L1 L21 A20 A9 A10 | A9 A14 L3 A15 | A14 L0 L1 | A9 A20 L3 A14 | A20 L21 A21 A9 | A21 L21 L15 L16 A319 L25 A320 A321 L27 L3 L9 L8 A9 | A9 A21 A11 L3 A20 | L1 L2 A20 L16 L13 L22 | A11 A317 L8 A316 A315 L3 | L8 A317 A11 | A315 A316 L8 L9 L3 | A20 L3 L12 L11 L10 | L10 A21 L3 A20 | L2 L3 A20 | A20 L3 A21 L16 | L10 L3 A21 | L27 A321 A322 L26 L28 L3 | L3 L28 L26 A323 A21 | A21 A323 L26 A322 A321 A320 L25 A319 | A22 | A3 | A16 | A17
sketch "Sketch2" plane through (0, 0, 0) normal (0, 0, 1) x (1, 0, 0)
  line L0 (23.2, 0) -> (0, 0)
  line L1 (0, 0) -> (0, -29.5)
  line L2 (0, -29.5) -> (23.2, -29.5)
  line L3 (23.2, -29.5) -> (23.2, 0)
  arc A0 (24.9891, -23.5483) -> (27.4891, -19.2182) centre (14.75, -14.75) ccw
  line L4 (27.4891, -19.2182) -> (23.4875, -16.9078)
  arc A1 (20.9875, -21.238) -> (23.4875, -16.9078) centre (14.75, -14.75) ccw construction
  line L5 (20.9875, -21.238) -> (24.9891, -23.5483)
  line L6 (6.0667, -12.4983) -> (1.9464, -10.2592)
  arc A2 (4.4591, -5.9072) -> (1.9464, -10.2592) centre (14.75, -14.75) ccw
  line L7 (4.4591, -5.9072) -> (8.5125, -8.262)
  line L8 (24.9891, -23.5483) -> (23.2, -23.5483)
  line L9 (20.9875, -21.238) -> (23.4875, -16.9078)
  line L10 (20.9875, -21.238) -> (23.2, -21.238)
  line L11 (8.5125, -8.262) -> (23.2, -8.262)
  line L12 (6.0667, -12.4983) -> (8.5125, -8.262)
  line L13 (4.4591, -5.9072) -> (23.2, -5.9072)
  circle A3 centre (14.75, -14.75) radius 5.5 projected
  circle A4 centre (14.75, -14.75) radius 14.75 projected
  circle A5 centre (14.75, -14.75) radius 14.25 projected
  circle A6 centre (14.75, -14.75) radius 5.5
  arc A7 (8.5125, -8.262) -> (6.0125, -12.5922) centre (14.75, -14.75) ccw construction
  line L14 (23.2, -23.5483) -> (27.5, -23.5483)
  line L15 (27.5, -23.5483) -> (27.5, -21.238)
  line L16 (27.5, -21.238) -> (23.2, -21.238)
  line L17 (23.2, -5.9072) -> (28.4, -5.9072)
  line L18 (28.4, -6.5) -> (28.4, 0) projected
  line L19 (23.2, -8.262) -> (28.4, -8.262)
  line L20 (28.4, -8.262) -> (28.4, -5.9072)
  line L21 (2.5, -1) -> (2.5, -17.5) projected
  line L22 (3, -7.965) -> (3, -10.8318)
  line L23 (26.7043, -21.0474) -> (25.0617, -19.4049) projected
  arc A8 (25.0617, -19.4049) -> (23.4815, -19.6245) centre (24.3546, -20.112) ccw projected
  arc A9 (19.6245, -23.4815) -> (23.4815, -19.6245) centre (14.75, -14.75) ccw projected
  arc A10 (19.6245, -23.4815) -> (19.4049, -25.0617) centre (20.112, -24.3546) ccw projected
  line L24 (19.4049, -25.0617) -> (21.0474, -26.7043) projected
  arc A11 (21.0474, -26.7043) -> (22.2832, -26.846) centre (21.7545, -25.9972) ccw projected
  arc A12 (2.654, -7.2168) -> (22.2832, -26.846) centre (14.75, -14.75) ccw projected
  arc A13 (2.654, -7.2168) -> (2.7957, -8.4526) centre (3.5028, -7.7455) ccw projected
  line L25 (2.7957, -8.4526) -> (4.4383, -10.0951) projected
  arc A14 (4.4383, -10.0951) -> (6.0185, -9.8755) centre (5.1454, -9.388) ccw projected
  arc A15 (9.8755, -6.0185) -> (6.0185, -9.8755) centre (14.75, -14.75) ccw projected
  arc A16 (9.8755, -6.0185) -> (10.0951, -4.4383) centre (9.388, -5.1454) ccw projected
  line L26 (10.0951, -4.4383) -> (8.4526, -2.7957) projected
  arc A17 (8.4526, -2.7957) -> (7.2168, -2.654) centre (7.7455, -3.5028) ccw projected
  arc A18 (26.846, -22.2832) -> (7.2168, -2.654) centre (14.75, -14.75) ccw projected
  arc A19 (26.846, -22.2832) -> (26.7043, -21.0474) centre (25.9972, -21.7545) ccw projected
  point P0 (0, 0)
  point P1 (23.1, -26.5191)
  point P2 (23.1, -18.8574)
  point P3 (6.8877, -8.4575)
  point P4 (5.3877, -11.0556)
  point P5 (24.0123, -18.3444)
  point P6 (22.5123, -20.9425)
  point P7 (6.0397, -9.7)
  point P8 (23.1, -20.0436)
  point P9 (23.1, -26.5191)
  point P10 (23.2, -22.5154)
  point P11 (23.2, -17.4058)
  point P12 (7.6168, -7.7416)
  point P13 (10.0358, -5.9072)
  point P14 (7.2168, -2.654)
  point P15 (2.654, -7.2168)
  point P16 (23.2, -20.0977)
  point P17 (22.2832, -26.846)
  point P18 (23.2, -26.2243)
  dimension "d34" = 6.3
  dimension "d157" = 2
  dimension "d205" = 0.5
  constraints: 42 end point, 9 point on circle, 7 perpendicular, 7 point on line, 5 centre point, 5 coincident, 5 parallel, 4 tangent, 3 horizontal, 1 collinear, 2 other
  measures "d34" distance edge to line of A4 L3
  measures "d157" distance edge to line of A4 L15
  measures "d205" distance between parallel lines of L22 L21
extrude "Extrusion5" cut sketch "Sketch2" against normal blind 4 contours L17 L18 L20 L19 A4 | A4 L19 A5 L17 | L17 A5 L19 L3 | L3 L11 L7 A15 A16 L13 | A17 L26 A16 L13 A2 A13 A5 | A11 L24 A10 A9 L5 L3 A5 | A16 A15 L7 L13 | A2 L22 L25 A13 | L7 A15 A14 L25 L22 A2 | L3 L10 A9 | L5 A9 L10 L3 | A3
sketch "Sketch3" plane through (28.4, 0, -9.3) normal (0, 0, -1) x (-1, 0, 0)
  circle A0 centre (19.3069, -61.8357) radius 1.0564
  circle A1 centre (7.9931, -50.522) radius 1.0564
  circle A2 centre (13.65, -56.1789) radius 14.75
  circle A3 centre (13.65, -14.75) radius 14.75
  line L0 (5.25, -66.4289) -> (28.4, -66.4289)
  line L1 (28.4, -66.4289) -> (28.4, 0)
  line L2 (28.4, 0) -> (4.3, 0)
  line L3 (0, -6.5) -> (0, 0)
  line L4 (0, -6.5) -> (0, 0) projected
  line L5 (0, 0) -> (28.4, 0) projected
  line L6 (4.3, 0) -> (0, 0)
  line L7 (26.9, -1) -> (26.9, -17)
  line L8 (25.9, -1) -> (26.9, -1)
  line L9 (25.9, -17) -> (25.9, -1)
  line L10 (25.9, -17) -> (26.9, -17)
  line L11 (28.4, -19.5) -> (5.3, -19.5)
  line L12 (5.3, -19.5) -> (0, -19.5)
  line L13 (0, -19.5) -> (0, -6.5) construction
  line L14 (0, -19.5) -> (0, -13.5)
  line L15 (0, -13.5) -> (25.9, -13.5)
  line L16 (25.9, -13.5) -> (25.9, -17.5)
  line L17 (25.9, -17.5) -> (27.4, -17.5)
  line L18 (27.4, -17.5) -> (27.4, -15)
  line L19 (27.4, -15) -> (28.4, -15)
  line L20 (28.4, -3.5) -> (27.4, -3.5)
  line L21 (27.4, -3.5) -> (27.4, -1)
  line L22 (27.4, -1) -> (25.9, -1)
  line L23 (25.9, -1) -> (25.9, -6.5)
  line L24 (5.2, -6.5) -> (0, -6.5) projected
  line L25 (25.9, -6.5) -> (0, -6.5)
  circle A4 centre (7.9931, -50.522) radius 2.25
  circle A5 centre (19.3069, -61.8357) radius 2.25
  line L26 (26.9, -1) -> (26.9, -17) projected
  line L27 (25.9, -1) -> (26.9, -1) projected
  line L28 (25.9, -17) -> (25.9, -1) projected
  line L29 (25.9, -17) -> (26.9, -17) projected
  circle A6 centre (13.65, -14.75) radius 14.75 projected
  circle A7 centre (13.65, -14.75) radius 14.25 projected
  circle A8 centre (13.65, -56.1789) radius 14.75 projected
  circle A9 centre (13.65, -56.1789) radius 14.25 projected
  circle A10 centre (19.3069, -61.8357) radius 1.0564 projected
  circle A11 centre (7.9931, -50.522) radius 1.0564 projected
  circle A12 centre (13.65, -56.1789) radius 5.5 projected
  circle A13 centre (13.65, -56.1789) radius 14.25 projected
  dimension "d81" = 4.5
  dimension "d83" = 2.5
  dimension "d84" = 6
  dimension "d85" = 0.5
  dimension "d86" = 2.5
  dimension "d87" = 0.5
  dimension "d88" = 0
  dimension "d89" = 2.5
  dimension "d90" = 0.5
  dimension "d91" = 0
  dimension "d92" = 0
  dimension "d95" = 4.5
  dimension "d96" = 4.5
  constraints: 46 end point, 8 perpendicular, 6 centre point, 6 coincident, 5 point on line, 5 tangent, 4 horizontal, 3 vertical, 1 collinear, 1 parallel
  measures "d81" distance edge to line of A2 L0
  measures "d83" distance between parallel lines of L11 L10
  measures "d84" distance between parallel lines of L11 L15
  measures "d85" distance between parallel lines of L18 L7
  measures "d86" distance between parallel lines of L17 L19
  measures "d87" distance between parallel lines of L17 L10
  measures "d88" distance between parallel lines of L9 L16
  measures "d89" distance between parallel lines of L22 L20
  measures "d90" distance between parallel lines of L7 L21
  measures "d91" distance between parallel lines of L22 L8
  measures "d92" distance between parallel lines of L9 L23
  measures "d95" diameter of A4
  measures "d96" diameter of A5
ref_plane "Work Plane3" through (1, -19, -16) normal (0, 0, 1) x (1, 0, 0)
extrude "Extrusion9" cut sketch "Sketch3" against normal blind 5.3 contours A0 | A1 | A4 | A5
ref_plane "Work Plane4" through (-5.099, -75.4361, 0) normal (0, 0, -1) x (0.7071068, 0.7071068, 0)
extrude "Extrusion10" cut sketch "Sketch3" against normal up to surface (9.3 mm away) contours A0 | A1
sketch "Sketch4" plane through (0, -66.4289, 0) normal (0, -1, 0) x (1, 0, 0)
  line L0 (0, 0) -> (23.2, 0) projected
  line L1 (0, 0) -> (0, -9.3) projected
  line L2 (0, -9.3) -> (23.2, -9.3) projected
  line L3 (23.2, 0) -> (23.2, -9.3) projected
  line L4 (4, 0) -> (4, -9.3)
  circle A0 centre (20.2, -6.8) radius 3
  circle A1 centre (14.2209, -6.3) radius 3
  circle A2 centre (14.2209, -6.3) radius 2.25
  circle A3 centre (20.2, -6.8) radius 2.5
  line L5 (0, 0) -> (23.2, 0) projected
  line L6 (11.3431, -9.3) -> (6.8431, -9.3) projected
  line L7 (6.8431, -9.3) -> (6.8431, 0)
  line L8 (0, -9.3) -> (23.2, -9.3) projected
  line L9 (23.2, 0) -> (23.2, -9.3) projected
  circle A4 centre (7, -6.3) radius 3
  dimension "d104" = 4
  dimension "d105" = 6
  dimension "d106" = 6
  dimension "d107" = 4.5
  dimension "d108" = 5
  dimension "d116" = 6
  constraints: 6 tangent, 5 centre point, 4 end point, 3 point on line, 2 coincident, 2 perpendicular
  measures "d104" distance between parallel lines of L1 L4
  measures "d105" diameter of A0
  measures "d106" diameter of A1
  measures "d107" diameter of A2
  measures "d108" diameter of A3
  measures "d116" diameter of A4
hole "Hole1" at (20.2, -66.4289, -6.8) direction (0, 1, 0) diameter 2.459 depth 13.25 thread size "M3x0.5" class "6H" standard "ISO Metric profile"
hole "Hole2" at (7, -66.4289, -6.3) at (14.2209, -66.4289, -6.3) direction (0, 1, 0) diameter 2.459 depth 8 thread size "M3x0.5" class "6H" standard "ISO Metric profile"